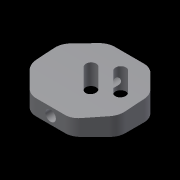
# Autodesk Inventor part: MiddleRouter
Saved by Autodesk Inventor 2015 (Build 190159000, 159)
## iProperties
Created: 2014-11-12
Part Number: MiddleRouter
Material: Generic
Document SubType Name: Modeling
Designer: Inventor
Density: 1 g/cm^3
Appearance: Default
Mass: 0.646659 g
Surface Area: 7.44519 cm^2
Volume: 0.646659 cm^3
Author: Inventor
Autodesk Inventor part; units mm, degrees
ref_plane "YZ Plane" through (0, 0, 0) normal (1, 0, 0) x (0, 1, 0)
ref_plane "XZ Plane" through (0, 0, 0) normal (0, 1, 0) x (-1, 0, 0)
ref_plane "XY Plane" through (0, 0, 0) normal (0, 0, 1) x (1, 0, 0)
sketch "Base" plane through (0, 0, 0) normal (0, 0, 1) x (1, 0, 0)
  line L0 (-8.5, -3) -> (-8.5, 3)
  line L1 (-8.5, 3) -> (-4, 7.5)
  line L2 (-4, 7.5) -> (4, 7.5)
  line L3 (4, 7.5) -> (8.5, 3)
  line L4 (8.5, 3) -> (8.5, -3)
  line L5 (8.5, -3) -> (4, -7.5)
  line L6 (4, -7.5) -> (-4, -7.5)
  line L7 (-4, -7.5) -> (-8.5, -3)
  line L8 (-8.5, 0) -> (8.5, 0) construction
  line L9 (0, 7.5) -> (0, -7.5) construction
  point P0 (0, 0)
  point P1 (0, 0)
  dimension "d1" = 17
  dimension "d5" = 15
  dimension "d7" = 6
  constraints: 20 end point, 7 midpoint, 4 parallel, 3 perpendicular, 2 vertical, 1 coincident, 1 horizontal
  measures "d1" distance between parallel lines of L4 L0
  measures "d5" distance between parallel lines of L6 L2
  measures "d7" distance of L3.end L4.end
extrude "BaseFeature" add sketch "Base" along normal blind 4
fillet "BaseFilletsFeature" radius 3 8 edges at (-8.5, -3, 2) (-4, -7.5, 2) (4, -7.5, 2) (8.5, -3, 2) (8.5, 3, 2) (4, 7.5, 2) (-4, 7.5, 2) (-8.5, 3, 2)
sketch "RailHoles" plane through (0, 0, 4) normal (0, 0, 1) x (1, 0, 0)
  line L0 (1.6663, 4.1769) -> (5.1769, 0.6663) construction
  line L1 (-1.8568, 2.0431) -> (1.6538, -1.4675) construction
  line L2 (7.6213, 3.8787) -> (4.8787, 6.6213) construction
  line L3 (6.25, 5.25) -> (3.4216, 2.4216) construction
  circle A0 centre (1.6663, 4.1769) radius 1
  circle A1 centre (5.1769, 0.6663) radius 1
  circle A2 centre (-1.8568, 2.0431) radius 1
  circle A3 centre (1.6538, -1.4675) radius 1
  line L4 (2.3734, 4.884) -> (5.884, 1.3734)
  line L5 (0.9592, 3.4698) -> (4.4698, -0.0408)
  line L6 (-1.1497, 2.7502) -> (2.3609, -0.7604)
  line L7 (-2.5639, 1.336) -> (0.9467, -2.1746)
  dimension "d11" = 4
  dimension "d12" = 4
  dimension "d13" = 4.9647
  dimension "d14" = 2
  dimension "d15" = 1.5
  dimension "d25" = 3.8787
  constraints: 14 end point, 8 point on circle, 8 tangent, 4 centre point, 4 coincident, 3 equal radius, 3 parallel, 2 midpoint, 1 perpendicular
  measures "d11" distance between parallel lines of L2 L0
  measures "d12" distance between parallel lines of L0 L1
  measures "d13" distance of L0.start L0.end
  measures "d14" diameter of A0
  measures "d15" distance from line of L1.end L3
  measures "d25" distance of L2.start L2.end
extrude "RailHolesFeature" cut sketch "RailHoles" against normal through all
sketch "RouteHole" plane through (-2.7574, -7.5, 0) normal (0, -1, 0) x (1, 0, 0)
  line L0 (5.5147, 4) -> (5.5147, 0) construction
  line L1 (0, 4) -> (5.5147, 4) construction
  line L2 (0, 0) -> (0, 4) construction
  line L3 (5.5147, 0) -> (0, 0) construction
  line L4 (0, 4) -> (0, 0) construction
  line L5 (0, 4) -> (5.5147, 4) construction
  line L6 (2.7574, 4) -> (2.7574, 0) construction
  line L7 (5.5147, 0) -> (0, 0) construction
  circle A0 centre (2.7574, 1.5) radius 1.25
  dimension "d40" = 2.5
  dimension "d41" = 1.5
  constraints: 2 end point, 2 midpoint, 1 centre point, 1 point on line
  measures "d40" diameter of A0
  measures "d41" distance from line of L3 A0.centre
hole "RouteHoleFeature" at (0, -7.5, 1.5) direction (0, 1, 0) diameter 2 end through all
sketch "SideProfile" plane through (8.5, -1.7574, 0) normal (1, 0, 0) x (0, 0, -1)
  arc A0 (-4, 9.2574) -> (-3, -5.7426) centre (109, 9.2574) ccw
  line L0 (-4, -5.7426) -> (0, -5.7426) construction
  line L1 (0, 9.2574) -> (-4, 9.2574) construction
  line L2 (-3, -5.7426) -> (0, -5.7426)
  line L3 (0, 9.2574) -> (0, -5.7426)
  line L4 (0, 9.2574) -> (0, 8.3787) projected
  line L5 (0, 9.2574) -> (-4, 9.2574)
  line L6 (-4, -2.1213) -> (-4, 0) construction
  dimension "d36" = 4
  dimension "d39" = 3
  constraints: 6 end point, 2 collinear, 2 point on circle, 2 point on line, 1 centre point, 1 perpendicular, 1 tangent
  measures "d36" distance of L1.start L5.end
  measures "d39" distance of L0.end L2.start
extrude "SideProfileFeature" cut sketch "SideProfile" against normal through all keep common part
equation "\"d7\" = 0.4 * d5"
equation "\"d12\" = 2 * d14"
equation "\"d13\" = 1.28 * d25"
